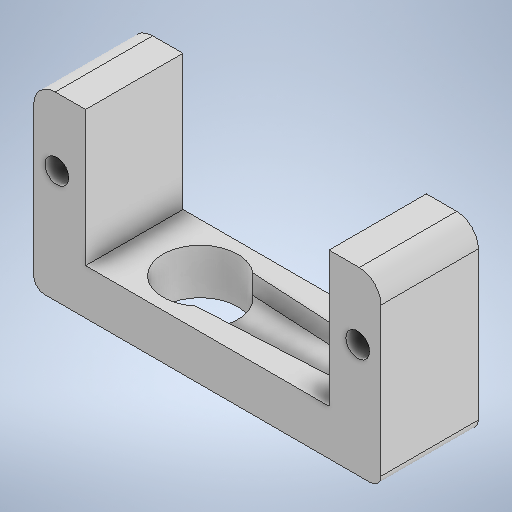
# Autodesk Inventor part: Hip v0.1
Saved by Autodesk Inventor 2025 (Build 290162000, 162)
## iProperties
Created: 2024-06-04
Part Number: Hip v0.1
Material: Generic
Document SubType Name: Modeling
Designer: sgols
Density: 1 g/cm^3
Appearance: Default
Mass: 1.86846 g
Surface Area: 17.0302 cm^2
Volume: 1.86846 cm^3
Author: sgols
Autodesk Inventor part; units mm, degrees
ref_plane "YZ Plane" through (0, 0, 0) normal (1, 0, 0) x (0, 1, 0)
ref_plane "XZ Plane" through (0, 0, 0) normal (0, 1, 0) x (-1, 0, 0)
sketch "Sketch1" plane through (0, 0, 0) normal (0, 0, 1) x (1, 0, 0)
  line L0 (-1.0988, -7.8697) -> (31.0012, -7.8697)
  line L1 (31.0012, -7.8697) -> (31.0012, 8.8303)
  line L2 (31.0012, 8.8303) -> (26.2012, 8.8303)
  line L3 (26.2012, 8.8303) -> (26.2012, -3.6697)
  line L4 (26.2012, -3.6697) -> (3.7012, -3.6697)
  line L5 (3.7012, -3.6697) -> (3.7012, 8.8303)
  line L6 (3.7012, 8.8303) -> (-1.0988, 8.8303)
  line L7 (-1.0988, 8.8303) -> (-1.0988, -7.8697)
  dimension "d5" = 4.8
  dimension "d6" = 22.5
  dimension "d7" = 12.5
  dimension "d8" = 4.2
  constraints: 16 end point, 3 perpendicular, 2 parallel, 2 point on line, 1 collinear, 1 horizontal, 1 vertical
  measures "d5" distance of L5.end L6.end
  measures "d6" distance of L3.end L4.end
  measures "d7" distance of L2.end L3.end
  measures "d8" distance between parallel lines of L0 L4
extrude "Extrusion1" add sketch "Sketch1" along normal mid plane 9
sketch "Sketch2" plane through (0, 0, 4.5) normal (0, 0, 1) x (1, 0, 0)
  line L0 (3.7012, -3.6697) -> (3.7012, 8.8303) projected
  line L1 (3.7012, 8.8303) -> (-1.0988, 8.8303) projected
  point P0 (0, 0)
  point P1 (3.7012, 2.5803)
  point P2 (3.7012, 2.5803)
  point P3 (1.0512, 2.5803)
  point P4 (3.7012, 2.5803)
  point P5 (3.7012, 2.5803)
  dimension "d14" = 2.65
  constraints: 4 midpoint, 1 horizontal alignment
  measures "d14" distance of point (3.701, 2.58) point (1.051, 2.58)
hole "Hole1" at (1.0512, 2.5803, 4.5) direction (0, 0, -1) diameter 2.2 end through all
ref_plane "Work Plane1" through (14.9512, -3.6697, 4.5) normal (-1, 0, 0) x (0, 0, 1)
mirror "Mirror1" about plane through (14.9512, -3.6697, 4.5) normal (-1, 0, 0) of "Hole1"
sketch "Sketch4" plane through (3.7012, -3.6697, 4.5) normal (0, 1, 0) x (1, 0, 0)
  line L0 (0, 9) -> (0, 0) projected
  line L1 (22.5, 0) -> (0, 0) projected
  line L2 (22.5, 9) -> (22.5, 0) projected
  line L3 (0, 9) -> (22.5, 9) projected
  circle A0 centre (6.1, 4.5) radius 3.45
  line L4 (8.3091, 7.15) -> (8.3091, 1.85) construction
  arc A1 (20.2591, 2.503) -> (20.2591, 6.497) centre (20.15, 4.5) ccw
  line L5 (8.3091, 7.15) -> (20.2591, 6.497)
  line L6 (8.3091, 1.85) -> (20.2591, 2.503)
  line L7 (6.1, 4.5) -> (20.15, 4.5) construction
  line L8 (0, 9) -> (0, 0) projected
  line L9 (0, 9) -> (0, 0) projected
  point P0 (-3.7012, 4.5)
  point P1 (11.25, 9)
  point P2 (0, 4.5)
  point P3 (0, 4.5)
  dimension "d23" = 5.3
  dimension "d25" = 2
  dimension "d26" = 14.05
  dimension "d27" = 6.9
  dimension "d28" = 6.1
  constraints: 8 end point, 4 point on circle, 3 midpoint, 2 centre point, 2 coincident, 2 tangent, 1 horizontal, 1 horizontal alignment, 1 vertical
  measures "d23" distance of L4.start L4.end
  measures "d25" radius of A1
  measures "d26" distance of L7.start L7.end
  measures "d27" diameter of A0
  measures "d28" distance from line of L9 L7.start
extrude "Extrusion2" cut sketch "Sketch4" against normal through all contours A0
extrude "Extrusion3" cut sketch "Sketch4" against normal blind 1.8 contours A0 L5 A1 L6
fillet "Fillet1" radius 2 2 edges at (-1.0988, 8.8303, 0) (31.0012, 8.8303, 0)
fillet "Fillet1" radius 1 2 edges at (31.0012, -7.8697, 0) (-1.0988, -7.8697, 0)
body "Solid1"
